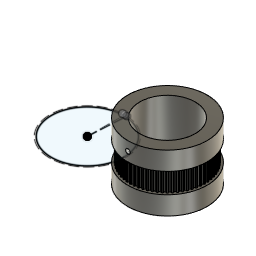
engranaje_gt2_parametrico_torreta (Autodesk Fusion 360 design; units mm, degrees)
Autodesk Fusion 360 part; units mm, degrees
(part 1 of 2)
sketch "Boceto1" plane through (0, 0, 0) normal (0, 0, 1) x (1, 0, 0)
  circle A0 centre (0, 0) radius 20.3718 construction
  line L0 (0, 0) -> (0, 19.6218) construction
  line L1 (0, 0) -> (0.9996, 20.3473) construction
  line L2 (0, 0) -> (1.3989, 20.3237) construction
  arc A1 (0.4973, 19.8971) -> (0.9628, 19.5982) centre (0.99, 20.1525) ccw
  arc A2 (0.2554, 20.3702) -> (0, 20.3718) centre (0, 0) ccw
  arc A3 (0.403, 20.2337) -> (0.2554, 20.3702) centre (0.2536, 20.2202) ccw
  arc A4 (0.403, 20.2337) -> (0.444, 20.0269) centre (1.3989, 20.3237) ccw
  arc A5 (0.444, 20.0269) -> (0.4973, 19.8971) centre (1.2025, 20.2627) ccw
  arc A6 (0, 20.3718) -> (-0.2554, 20.3702) centre (0, 0) ccw
  arc A7 (-0.2554, 20.3702) -> (-0.403, 20.2337) centre (-0.2536, 20.2202) ccw
  arc A8 (-0.444, 20.0269) -> (-0.403, 20.2337) centre (-1.3989, 20.3237) ccw
  arc A9 (-0.4973, 19.8971) -> (-0.444, 20.0269) centre (-1.2025, 20.2627) ccw
  arc A10 (-0.9628, 19.5982) -> (-0.4973, 19.8971) centre (-0.99, 20.1525) ccw
  arc A11 (0.9628, 19.5982) -> (-0.9628, 19.5982) centre (0, 0) ccw construction
  arc A12 (0.9628, 19.5982) -> (-0.9628, 19.5982) centre (0, 0) ccw
  circle A13 centre (0, 0) radius 19.6218
  dimension "d21" = 2.812
  dimension "d22" = 1.125
  dimension "d23" = 0.75
  dimension "d24" = 40.7437
  dimension "d25" = 0.555
  dimension "d26" = 2
  dimension "d27" = 0.3
  dimension "d31" = 0.75
  constraint coincident A0.centre L0.start
  constraint coincident L0.end A11
  constraint vertical L0
  constraint coincident A0 L1.end
  constraint coincident A0 L2.end
  constraint coincident L1 A1.end
  constraint coincident L1 A1.centre
  constraint coincident L2.end A4.centre
  constraint tangent A3 A4
  constraint tangent A0 A3
  constraint coincident A0 A2.end
  constraint tangent A4 A5
  constraint tangent A1 A5
  constraint symmetric L0 A1.start A9.start
  constraint symmetric L0 A1.end A10.start
  constraint symmetric L0 A1 A10
  constraint symmetric L0 A2.start A6.end
  constraint symmetric L0 A2.end A6.start
  constraint symmetric L0 A2 A6
  constraint symmetric L0 A3.start A7.end
  constraint symmetric L0 A3 A7
  constraint symmetric L0 A4.end A8.start
  constraint symmetric L0 A4 A8
  constraint symmetric L0 A5 A9
  constraint concentric A0 A12
  constraint coincident L0.end A12
  constraint concentric A12 A13
  measures "d21" angle of L0 L1
  measures "d22" angle of L1 L2
  measures "d23" distance of A0 A11
  measures "d24" diameter of A0
  measures "d25" radius of A1
  measures "d26" diameter of A4
  measures "d27" diameter of A3
  measures "d31" distance of A0 A13
sketch "Boceto5" plane through (0, 0, 0) normal (0, 0, 1) x (1, 0, 0)
sketch "Boceto6" plane through (0, 0, 0) normal (0, 0, 1) x (1, 0, 0)
sketch "Boceto7" plane through (0, 0, 0) normal (0, 0, 1) x (1, 0, 0)
extrude "Extruir8" add sketch "Boceto1" along normal blind 11 contours A1 A2 A3 A4 A5 A6 A7 A8 A9 A10 A12 A13 makes body 1
pattern_circular "Patrón C3" count 64 over 360 about axis through (0, 0, 1.75) along (0, 0, 1) of bodies 1 makes body 2 at (-2.6672, 19.4397, 7.3333) makes body 3 at (-4.5598, 19.0847, 7.3333) makes body 4 at (-6.4085, 18.5458, 7.3333) makes body 5 at (-7.6077, 18.087, 7.3333) makes body 6 at (-9.3439, 17.2542, 7.3333) makes body 7 at (-10.2706, 16.7192, 3.6667) makes body 8 at (-13.0178, 14.6817, 7.3333) makes body 9 at (-14.3942, 13.335, 7.3333) makes body 10 at (-15.632, 11.8599, 7.3333) makes body 11 at (-15.887, 11.5161, 3.6667) makes body 12 at (-17.5507, 8.7744, 7.3333) makes body 13 at (-18.1689, 7.41, 7.3333) makes body 14 at (-18.5458, 6.4085, 3.6667) makes body 15 at (-19.3769, 3.0907, 7.3333) makes body 16 at (-19.5865, 1.1765, 7.3333) makes body 17 at (-19.6075, 0.749, 3.6667) makes body 18 at (-19.4397, -2.6672, 7.3333) makes body 19 at (-19.3769, -3.0907, 3.6667) makes body 20 at (-18.7456, -5.7982, 7.3333) makes body 21 at (-18.087, -7.6077, 7.3333) makes body 22 at (-16.9392, -9.9035, 7.3333) makes body 23 at (-16.2553, -10.9901, 7.3333) makes body 24 at (-14.6817, -13.0178, 7.3333) makes body 25 at (-14.3942, -13.335, 3.6667) makes body 26 at (-11.8599, -15.632, 7.3333) makes body 27 at (-10.8122, -16.3742, 7.3333) makes body 28 at (-9.1551, -17.3551, 7.3333) makes body 29 at (-7.41, -18.1689, 7.3333) makes body 30 at (-6.4085, -18.5458, 3.6667) makes body 31 at (-3.0907, -19.3769, 7.3333) makes body 32 at (-1.1765, -19.5865, 7.3333) makes body 33 at (-0.749, -19.6075, 3.6667) makes body 34 at (2.6672, -19.4397, 7.3333) makes body 35 at (3.0907, -19.3769, 3.6667) makes body 36 at (6.4085, -18.5458, 7.3333) makes body 37 at (8.1954, -17.8284, 7.3333) makes body 38 at (8.5824, -17.6454, 3.6667) makes body 39 at (11.3421, -16.0116, 7.3333) makes body 40 at (13.0178, -14.6817, 7.3333) makes body 41 at (13.335, -14.3942, 3.6667) makes body 42 at (15.632, -11.8599, 7.3333) makes body 43 at (15.887, -11.5161, 3.6667) makes body 44 at (17.6454, -8.5824, 7.3333) makes body 45 at (18.1689, -7.41, 7.3333) makes body 46 at (18.5458, -6.4085, 3.6667) makes body 47 at (19.3769, -3.0907, 7.3333) makes body 48 at (19.5865, -1.1765, 7.3333) makes body 49 at (19.6075, 0.749, 7.3333) makes body 50 at (19.4397, 2.6672, 7.3333) makes body 51 at (19.3769, 3.0907, 3.6667) makes body 52 at (18.5458, 6.4085, 7.3333) makes body 53 at (18.087, 7.6077, 7.3333) makes body 54 at (17.2542, 9.3439, 7.3333) makes body 55 at (16.2553, 10.9901, 7.3333) makes body 56 at (14.6817, 13.0178, 7.3333) makes body 57 at (13.335, 14.3942, 7.3333) makes body 58 at (11.8599, 15.632, 7.3333) makes body 59 at (11.5161, 15.887, 3.6667) makes body 60 at (8.5824, 17.6454, 7.3333) makes body 61 at (7.41, 18.1689, 7.3333) makes body 62 at (6.4085, 18.5458, 3.6667) makes body 63 at (3.723, 19.2654, 7.3333) makes body 64 at (1.1765, 19.5865, 7.3333)
extrude "Extruir9" add sketch "Boceto1" along normal blind 11 contours A12 A13 bodies 1 2 3 4 5 6 7 8 9 10 11 12 13 14 15 16 17 18 19 20 21 22 23 24 25 26 27 28 29 30 31 32 33 34 35 36 37 38 39 40 41 42 43 44 45 46 47 48 49 50 51 52 53 54 55 56 57 58 59 60 61 62 63 64
sketch "Boceto8" plane through (0, 0, 11) normal (0, 0, 1) x (-1, 0, 0)
  arc A0 (0.403, 20.2337) -> (0.2554, 20.3702) centre (0.2536, 20.2202) ccw
  arc A1 (0.2554, 20.3702) -> (-0.2554, 20.3702) centre (0, 0) ccw
  arc A2 (-0.2554, 20.3702) -> (-0.403, 20.2337) centre (-0.2536, 20.2202) ccw
  arc A3 (-0.444, 20.0269) -> (-0.403, 20.2337) centre (-1.3989, 20.3237) ccw
  arc A4 (-0.4973, 19.8971) -> (-0.444, 20.0269) centre (-1.2025, 20.2627) ccw
  arc A5 (-0.9628, 19.5982) -> (-0.4973, 19.8971) centre (-0.99, 20.1525) ccw
  arc A6 (-1.4553, 19.85) -> (-0.9628, 19.5982) centre (-0.99, 20.1525) ccw
  arc A7 (-1.5211, 19.974) -> (-1.4553, 19.85) centre (-0.7893, 20.283) ccw
  arc A8 (-1.5822, 20.1758) -> (-1.5211, 19.974) centre (-0.5999, 20.363) ccw
  arc A9 (-1.5822, 20.1758) -> (-1.7424, 20.2972) centre (-1.7296, 20.1477) ccw
  arc A10 (-1.7424, 20.2972) -> (-2.2508, 20.2471) centre (0, 0) ccw
  arc A11 (-2.2508, 20.2471) -> (-2.3843, 20.0968) centre (-2.2343, 20.098) ccw
  arc A12 (-2.4048, 19.887) -> (-2.3843, 20.0968) centre (-3.3842, 20.0888) ccw
  arc A13 (-2.4452, 19.7525) -> (-2.4048, 19.887) centre (-3.1828, 20.0473) ccw
  arc A14 (-2.8791, 19.4095) -> (-2.4452, 19.7525) centre (-2.9606, 19.9584) ccw
  arc A15 (-3.394, 19.6118) -> (-2.8791, 19.4095) centre (-2.9606, 19.9584) ccw
  arc A16 (-3.4716, 19.7287) -> (-3.394, 19.6118) centre (-2.7736, 20.108) ccw
  arc A17 (-3.5522, 19.9236) -> (-3.4716, 19.7287) centre (-2.5929, 20.2061) ccw
  arc A18 (-3.5522, 19.9236) -> (-3.7235, 20.0287) centre (-3.6961, 19.8812) ccw
  arc A19 (-3.7235, 20.0287) -> (-4.2245, 19.929) centre (0, 0) ccw
  arc A20 (-4.2245, 19.929) -> (-4.3426, 19.7663) centre (-4.1935, 19.7822) ccw
  arc A21 (-4.3425, 19.5555) -> (-4.3426, 19.7663) centre (-5.337, 19.6603) ccw
  arc A22 (-4.3695, 19.4177) -> (-4.3425, 19.5555) centre (-5.1325, 19.6388) ccw
  arc A23 (-4.7677, 19.0338) -> (-4.3695, 19.4177) centre (-4.9026, 19.5722) ccw
  arc A24 (-5.2999, 19.1847) -> (-4.7677, 19.0338) centre (-4.9026, 19.5722) ccw
  arc A25 (-5.3886, 19.2934) -> (-5.2999, 19.1847) centre (-4.7312, 19.7393) ccw
  arc A26 (-5.4879, 19.4795) -> (-5.3886, 19.2934) centre (-4.561, 19.8547) ccw
  arc A27 (-5.4879, 19.4795) -> (-5.6687, 19.5672) centre (-5.627, 19.4232) ccw
  arc A28 (-5.6687, 19.5672) -> (-6.1576, 19.419) centre (0, 0) ccw
  arc A29 (-6.1576, 19.419) -> (-6.2592, 19.2455) centre (-6.1123, 19.276) ccw
  arc A30 (-6.2384, 19.0357) -> (-6.2592, 19.2455) centre (-7.2383, 19.0425) ccw
  arc A31 (-6.2517, 18.896) -> (-6.2384, 19.0357) centre (-7.0327, 19.0411) ccw
  arc A32 (-6.6104, 18.4748) -> (-6.2517, 18.896) centre (-6.7974, 18.9974) ccw
  arc A33 (-7.1548, 18.5728) -> (-6.6104, 18.4748) centre (-6.7974, 18.9974) ccw
  arc A34 (-7.2538, 18.6723) -> (-7.1548, 18.5728) centre (-6.6432, 19.1805) ccw
  arc A35 (-7.3708, 18.8477) -> (-7.2538, 18.6723) centre (-6.4851, 19.312) ccw
  arc A36 (-7.3708, 18.8477) -> (-7.5594, 18.9174) centre (-7.5037, 18.7781) ccw
  arc A37 (-7.5594, 18.9174) -> (-8.0313, 18.7219) centre (0, 0) ccw
  arc A38 (-8.0313, 18.7219) -> (-8.1154, 18.5393) centre (-7.9722, 18.584) ccw
  arc A39 (-8.0741, 18.3325) -> (-8.1154, 18.5393) centre (-9.07, 18.2414) ccw
  arc A40 (-8.0737, 18.1922) -> (-8.0741, 18.3325) centre (-8.8652, 18.2601) ccw
  arc A41 (-8.3894, 17.7379) -> (-8.0737, 18.1922) centre (-8.6267, 18.2396) ccw
  arc A42 (-8.9408, 17.7821) -> (-8.3894, 17.7379) centre (-8.6267, 18.2396) ccw
  arc A43 (-9.0491, 17.8714) -> (-8.9408, 17.7821) centre (-8.4912, 18.437) ccw
  arc A44 (-9.1827, 18.0345) -> (-9.0491, 17.8714) centre (-8.3468, 18.5834) ccw
  arc A45 (-9.1827, 18.0345) -> (-9.3772, 18.0853) centre (-9.3081, 17.9522) ccw
  arc A46 (-9.3772, 18.0853) -> (-9.8277, 17.8445) centre (0, 0) ccw
  arc A47 (-9.8277, 17.8445) -> (-9.8935, 17.6546) centre (-9.7554, 17.7131) ccw
  arc A48 (-9.8322, 17.4529) -> (-9.8935, 17.6546) centre (-10.8143, 17.2645) ccw
  arc A49 (-9.818, 17.3132) -> (-9.8322, 17.4529) centre (-10.6123, 17.3032) ccw
  arc A50 (-10.0876, 16.8302) -> (-9.818, 17.3132) centre (-10.373, 17.3062) ccw
  arc A51 (-10.6407, 16.8201) -> (-10.0876, 16.8302) centre (-10.373, 17.3062) ccw
  arc A52 (-10.7572, 16.8984) -> (-10.6407, 16.8201) centre (-10.2575, 17.5159) ccw
  arc A53 (-10.9062, 17.0476) -> (-10.7572, 16.8984) centre (-10.1281, 17.6758) ccw
  arc A54 (-10.9062, 17.0476) -> (-11.1047, 17.0791) centre (-11.0229, 16.9534) ccw
  arc A55 (-11.1047, 17.0791) -> (-11.5295, 16.7953) centre (0, 0) ccw
  arc A56 (-11.5295, 16.7953) -> (-11.5763, 16.5999) centre (-11.4446, 16.6716) ccw
  arc A57 (-11.4955, 16.4051) -> (-11.5763, 16.5999) centre (-12.4544, 16.1214) ccw
  arc A58 (-11.4677, 16.2675) -> (-11.4955, 16.4051) centre (-12.2572, 16.1797) ccw
  arc A59 (-11.6887, 15.7604) -> (-11.4677, 16.2675) centre (-12.0193, 16.2062) ccw
  arc A60 (-12.2381, 15.6961) -> (-11.6887, 15.7604) centre (-12.0193, 16.2062) ccw
  arc A61 (-12.3617, 15.7627) -> (-12.2381, 15.6961) centre (-11.9249, 16.4262) ccw
  arc A62 (-12.5247, 15.8965) -> (-12.3617, 15.7627) centre (-11.8119, 16.5979) ccw
  arc A63 (-12.5247, 15.8965) -> (-12.7253, 15.9084) centre (-12.6316, 15.7913) ccw
  arc A64 (-12.7253, 15.9084) -> (-13.1202, 15.5844) centre (0, 0) ccw
  arc A65 (-13.1202, 15.5844) -> (-13.1476, 15.3853) centre (-13.0236, 15.4696) ccw
  arc A66 (-13.0481, 15.1994) -> (-13.1476, 15.3853) centre (-13.9746, 14.823) ccw
  arc A67 (-13.007, 15.0652) -> (-13.0481, 15.1994) centre (-13.7841, 14.9004) ccw
  arc A68 (-13.1772, 14.5388) -> (-13.007, 15.0652) centre (-13.5499, 14.95) ccw
  arc A69 (-13.7177, 14.421) -> (-13.1772, 14.5388) centre (-13.5499, 14.95) ccw
  arc A70 (-13.8472, 14.4751) -> (-13.7177, 14.421) centre (-13.4776, 15.1782) ccw
  arc A71 (-14.0225, 14.5924) -> (-13.8472, 14.4751) centre (-13.3819, 15.3602) ccw
  arc A72 (-14.0225, 14.5924) -> (-14.2233, 14.5845) centre (-14.1186, 14.4772) ccw
  arc A73 (-14.2233, 14.5845) -> (-14.5845, 14.2233) centre (0, 0) ccw
  arc A74 (-14.5845, 14.2233) -> (-14.5924, 14.0225) centre (-14.4772, 14.1186) ccw
  arc A75 (-14.4751, 13.8472) -> (-14.5924, 14.0225) centre (-15.3602, 13.3819) ccw
  arc A76 (-14.421, 13.7177) -> (-14.4751, 13.8472) centre (-15.1782, 13.4776) ccw
  arc A77 (-14.5388, 13.1772) -> (-14.421, 13.7177) centre (-14.95, 13.5499) ccw
  arc A78 (-15.0652, 13.007) -> (-14.5388, 13.1772) centre (-14.95, 13.5499) ccw
  arc A79 (-15.1994, 13.0481) -> (-15.0652, 13.007) centre (-14.9004, 13.7841) ccw
  arc A80 (-15.3853, 13.1476) -> (-15.1994, 13.0481) centre (-14.823, 13.9746) ccw
  arc A81 (-15.3853, 13.1476) -> (-15.5844, 13.1202) centre (-15.4696, 13.0236) ccw
  arc A82 (-15.5844, 13.1202) -> (-15.9084, 12.7253) centre (0, 0) ccw
  arc A83 (-15.9084, 12.7253) -> (-15.8965, 12.5247) centre (-15.7913, 12.6316) ccw
  arc A84 (-15.7627, 12.3617) -> (-15.8965, 12.5247) centre (-16.5979, 11.8119) ccw
  arc A85 (-15.6961, 12.2381) -> (-15.7627, 12.3617) centre (-16.4262, 11.9249) ccw
  arc A86 (-15.7604, 11.6887) -> (-15.6961, 12.2381) centre (-16.2062, 12.0193) ccw
  arc A87 (-16.2675, 11.4677) -> (-15.7604, 11.6887) centre (-16.2062, 12.0193) ccw
  arc A88 (-16.4051, 11.4955) -> (-16.2675, 11.4677) centre (-16.1797, 12.2572) ccw
  arc A89 (-16.5999, 11.5763) -> (-16.4051, 11.4955) centre (-16.1214, 12.4544) ccw
  arc A90 (-16.5999, 11.5763) -> (-16.7953, 11.5295) centre (-16.6716, 11.4446) ccw
  arc A91 (-16.7953, 11.5295) -> (-17.0791, 11.1047) centre (0, 0) ccw
  arc A92 (-17.0791, 11.1047) -> (-17.0476, 10.9062) centre (-16.9534, 11.0229) ccw
  arc A93 (-16.8984, 10.7572) -> (-17.0476, 10.9062) centre (-17.6758, 10.1281) ccw
  arc A94 (-16.8201, 10.6407) -> (-16.8984, 10.7572) centre (-17.5159, 10.2575) ccw
  arc A95 (-16.8302, 10.0876) -> (-16.8201, 10.6407) centre (-17.3062, 10.373) ccw
  arc A96 (-17.3132, 9.818) -> (-16.8302, 10.0876) centre (-17.3062, 10.373) ccw
  arc A97 (-17.4529, 9.8322) -> (-17.3132, 9.818) centre (-17.3032, 10.6123) ccw
  arc A98 (-17.6546, 9.8935) -> (-17.4529, 9.8322) centre (-17.2645, 10.8143) ccw
  arc A99 (-17.6546, 9.8935) -> (-17.8445, 9.8277) centre (-17.7131, 9.7554) ccw
  arc A100 (-17.8445, 9.8277) -> (-18.0853, 9.3772) centre (0, 0) ccw
  arc A101 (-18.0853, 9.3772) -> (-18.0345, 9.1827) centre (-17.9522, 9.3081) ccw
  arc A102 (-17.8714, 9.0491) -> (-18.0345, 9.1827) centre (-18.5834, 8.3468) ccw
  arc A103 (-17.7821, 8.9408) -> (-17.8714, 9.0491) centre (-18.437, 8.4912) ccw
  arc A104 (-17.7379, 8.3894) -> (-17.7821, 8.9408) centre (-18.2396, 8.6267) ccw
  arc A105 (-18.1922, 8.0737) -> (-17.7379, 8.3894) centre (-18.2396, 8.6267) ccw
  arc A106 (-18.3325, 8.0741) -> (-18.1922, 8.0737) centre (-18.2601, 8.8652) ccw
  arc A107 (-18.5393, 8.1154) -> (-18.3325, 8.0741) centre (-18.2414, 9.07) ccw
  arc A108 (-18.5393, 8.1154) -> (-18.7219, 8.0313) centre (-18.584, 7.9722) ccw
  arc A109 (-18.7219, 8.0313) -> (-18.9174, 7.5594) centre (0, 0) ccw
  arc A110 (-18.9174, 7.5594) -> (-18.8477, 7.3708) centre (-18.7781, 7.5037) ccw
  arc A111 (-18.6723, 7.2538) -> (-18.8477, 7.3708) centre (-19.312, 6.4851) ccw
  arc A112 (-18.5728, 7.1548) -> (-18.6723, 7.2538) centre (-19.1805, 6.6432) ccw
  arc A113 (-18.4748, 6.6104) -> (-18.5728, 7.1548) centre (-18.9974, 6.7974) ccw
  arc A114 (-18.896, 6.2517) -> (-18.4748, 6.6104) centre (-18.9974, 6.7974) ccw
  arc A115 (-19.0357, 6.2384) -> (-18.896, 6.2517) centre (-19.0411, 7.0327) ccw
  arc A116 (-19.2455, 6.2592) -> (-19.0357, 6.2384) centre (-19.0425, 7.2383) ccw
  arc A117 (-19.2455, 6.2592) -> (-19.419, 6.1576) centre (-19.276, 6.1123) ccw
  arc A118 (-19.419, 6.1576) -> (-19.5672, 5.6687) centre (0, 0) ccw
  arc A119 (-19.5672, 5.6687) -> (-19.4795, 5.4879) centre (-19.4232, 5.627) ccw
  arc A120 (-19.2934, 5.3886) -> (-19.4795, 5.4879) centre (-19.8547, 4.561) ccw
  arc A121 (-19.1847, 5.2999) -> (-19.2934, 5.3886) centre (-19.7393, 4.7312) ccw
  arc A122 (-19.0338, 4.7677) -> (-19.1847, 5.2999) centre (-19.5722, 4.9026) ccw
  arc A123 (-19.4177, 4.3695) -> (-19.0338, 4.7677) centre (-19.5722, 4.9026) ccw
  arc A124 (-19.5555, 4.3425) -> (-19.4177, 4.3695) centre (-19.6388, 5.1325) ccw
  arc A125 (-19.7663, 4.3426) -> (-19.5555, 4.3425) centre (-19.6603, 5.337) ccw
  arc A126 (-19.7663, 4.3426) -> (-19.929, 4.2245) centre (-19.7822, 4.1935) ccw
  arc A127 (-19.929, 4.2245) -> (-20.0287, 3.7235) centre (0, 0) ccw
  arc A128 (-20.0287, 3.7235) -> (-19.9236, 3.5522) centre (-19.8812, 3.6961) ccw
  arc A129 (-19.7287, 3.4716) -> (-19.9236, 3.5522) centre (-20.2061, 2.5929) ccw
  arc A130 (-19.6118, 3.394) -> (-19.7287, 3.4716) centre (-20.108, 2.7736) ccw
  arc A131 (-19.4095, 2.8791) -> (-19.6118, 3.394) centre (-19.9584, 2.9606) ccw
  arc A132 (-19.7525, 2.4452) -> (-19.4095, 2.8791) centre (-19.9584, 2.9606) ccw
  arc A133 (-19.887, 2.4048) -> (-19.7525, 2.4452) centre (-20.0473, 3.1828) ccw
  arc A134 (-20.0968, 2.3843) -> (-19.887, 2.4048) centre (-20.0888, 3.3842) ccw
  arc A135 (-20.0968, 2.3843) -> (-20.2471, 2.2508) centre (-20.098, 2.2343) ccw
  arc A136 (-20.2471, 2.2508) -> (-20.2972, 1.7424) centre (0, 0) ccw
  arc A137 (-20.2972, 1.7424) -> (-20.1758, 1.5822) centre (-20.1477, 1.7296) ccw
  arc A138 (-19.974, 1.5211) -> (-20.1758, 1.5822) centre (-20.363, 0.5999) ccw
  arc A139 (-19.85, 1.4553) -> (-19.974, 1.5211) centre (-20.283, 0.7893) ccw
  arc A140 (-19.5982, 0.9628) -> (-19.85, 1.4553) centre (-20.1525, 0.99) ccw
  arc A141 (-19.8971, 0.4973) -> (-19.5982, 0.9628) centre (-20.1525, 0.99) ccw
  arc A142 (-20.0269, 0.444) -> (-19.8971, 0.4973) centre (-20.2627, 1.2025) ccw
  arc A143 (-20.2337, 0.403) -> (-20.0269, 0.444) centre (-20.3237, 1.3989) ccw
  arc A144 (-20.2337, 0.403) -> (-20.3702, 0.2554) centre (-20.2202, 0.2536) ccw
  arc A145 (-20.3702, 0.2554) -> (-20.3702, -0.2554) centre (0, 0) ccw
  arc A146 (-20.3702, -0.2554) -> (-20.2337, -0.403) centre (-20.2202, -0.2536) ccw
  arc A147 (-20.0269, -0.444) -> (-20.2337, -0.403) centre (-20.3237, -1.3989) ccw
  arc A148 (-19.8971, -0.4973) -> (-20.0269, -0.444) centre (-20.2627, -1.2025) ccw
  arc A149 (-19.5982, -0.9628) -> (-19.8971, -0.4973) centre (-20.1525, -0.99) ccw
  arc A150 (-19.85, -1.4553) -> (-19.5982, -0.9628) centre (-20.1525, -0.99) ccw
  arc A151 (-19.974, -1.5211) -> (-19.85, -1.4553) centre (-20.283, -0.7893) ccw
  arc A152 (-20.1758, -1.5822) -> (-19.974, -1.5211) centre (-20.363, -0.5999) ccw
  arc A153 (-20.1758, -1.5822) -> (-20.2972, -1.7424) centre (-20.1477, -1.7296) ccw
  arc A154 (-20.2972, -1.7424) -> (-20.2471, -2.2508) centre (0, 0) ccw
  arc A155 (-20.2471, -2.2508) -> (-20.0968, -2.3843) centre (-20.098, -2.2343) ccw
  arc A156 (-19.887, -2.4048) -> (-20.0968, -2.3843) centre (-20.0888, -3.3842) ccw
  arc A157 (-19.7525, -2.4452) -> (-19.887, -2.4048) centre (-20.0473, -3.1828) ccw
  arc A158 (-19.4095, -2.8791) -> (-19.7525, -2.4452) centre (-19.9584, -2.9606) ccw
  arc A159 (-19.6118, -3.394) -> (-19.4095, -2.8791) centre (-19.9584, -2.9606) ccw
  arc A160 (-19.7287, -3.4716) -> (-19.6118, -3.394) centre (-20.108, -2.7736) ccw
  arc A161 (-19.9236, -3.5522) -> (-19.7287, -3.4716) centre (-20.2061, -2.5929) ccw
  arc A162 (-19.9236, -3.5522) -> (-20.0287, -3.7235) centre (-19.8812, -3.6961) ccw
  arc A163 (-20.0287, -3.7235) -> (-19.929, -4.2245) centre (0, 0) ccw
  arc A164 (-19.929, -4.2245) -> (-19.7663, -4.3426) centre (-19.7822, -4.1935) ccw
  arc A165 (-19.5555, -4.3425) -> (-19.7663, -4.3426) centre (-19.6603, -5.337) ccw
  arc A166 (-19.4177, -4.3695) -> (-19.5555, -4.3425) centre (-19.6388, -5.1325) ccw
  arc A167 (-19.0338, -4.7677) -> (-19.4177, -4.3695) centre (-19.5722, -4.9026) ccw
  arc A168 (-19.1847, -5.2999) -> (-19.0338, -4.7677) centre (-19.5722, -4.9026) ccw
  arc A169 (-19.2934, -5.3886) -> (-19.1847, -5.2999) centre (-19.7393, -4.7312) ccw
  arc A170 (-19.4795, -5.4879) -> (-19.2934, -5.3886) centre (-19.8547, -4.561) ccw
  arc A171 (-19.4795, -5.4879) -> (-19.5672, -5.6687) centre (-19.4232, -5.627) ccw
  arc A172 (-19.5672, -5.6687) -> (-19.419, -6.1576) centre (0, 0) ccw
  arc A173 (-19.419, -6.1576) -> (-19.2455, -6.2592) centre (-19.276, -6.1123) ccw
  arc A174 (-19.0357, -6.2384) -> (-19.2455, -6.2592) centre (-19.0425, -7.2383) ccw
  arc A175 (-18.896, -6.2517) -> (-19.0357, -6.2384) centre (-19.0411, -7.0327) ccw
  arc A176 (-18.4748, -6.6104) -> (-18.896, -6.2517) centre (-18.9974, -6.7974) ccw
  arc A177 (-18.5728, -7.1548) -> (-18.4748, -6.6104) centre (-18.9974, -6.7974) ccw
  arc A178 (-18.6723, -7.2538) -> (-18.5728, -7.1548) centre (-19.1805, -6.6432) ccw
  arc A179 (-18.8477, -7.3708) -> (-18.6723, -7.2538) centre (-19.312, -6.4851) ccw
  arc A180 (-18.8477, -7.3708) -> (-18.9174, -7.5594) centre (-18.7781, -7.5037) ccw
  arc A181 (-18.9174, -7.5594) -> (-18.7219, -8.0313) centre (0, 0) ccw
  arc A182 (-18.7219, -8.0313) -> (-18.5393, -8.1154) centre (-18.584, -7.9722) ccw
  arc A183 (-18.3325, -8.0741) -> (-18.5393, -8.1154) centre (-18.2414, -9.07) ccw
  arc A184 (-18.1922, -8.0737) -> (-18.3325, -8.0741) centre (-18.2601, -8.8652) ccw
  arc A185 (-17.7379, -8.3894) -> (-18.1922, -8.0737) centre (-18.2396, -8.6267) ccw
  arc A186 (-17.7821, -8.9408) -> (-17.7379, -8.3894) centre (-18.2396, -8.6267) ccw
  arc A187 (-17.8714, -9.0491) -> (-17.7821, -8.9408) centre (-18.437, -8.4912) ccw
  arc A188 (-18.0345, -9.1827) -> (-17.8714, -9.0491) centre (-18.5834, -8.3468) ccw
  arc A189 (-18.0345, -9.1827) -> (-18.0853, -9.3772) centre (-17.9522, -9.3081) ccw
  arc A190 (-18.0853, -9.3772) -> (-17.8445, -9.8277) centre (0, 0) ccw
  arc A191 (-17.8445, -9.8277) -> (-17.6546, -9.8935) centre (-17.7131, -9.7554) ccw
  arc A192 (-17.4529, -9.8322) -> (-17.6546, -9.8935) centre (-17.2645, -10.8143) ccw
  arc A193 (-17.3132, -9.818) -> (-17.4529, -9.8322) centre (-17.3032, -10.6123) ccw
  arc A194 (-16.8302, -10.0876) -> (-17.3132, -9.818) centre (-17.3062, -10.373) ccw
  arc A195 (-16.8201, -10.6407) -> (-16.8302, -10.0876) centre (-17.3062, -10.373) ccw
  arc A196 (-16.8984, -10.7572) -> (-16.8201, -10.6407) centre (-17.5159, -10.2575) ccw
  arc A197 (-17.0476, -10.9062) -> (-16.8984, -10.7572) centre (-17.6758, -10.1281) ccw
  arc A198 (-17.0476, -10.9062) -> (-17.0791, -11.1047) centre (-16.9534, -11.0229) ccw
  arc A199 (-17.0791, -11.1047) -> (-16.7953, -11.5295) centre (0, 0) ccw
  arc A200 (-16.7953, -11.5295) -> (-16.5999, -11.5763) centre (-16.6716, -11.4446) ccw
  arc A201 (-16.4051, -11.4955) -> (-16.5999, -11.5763) centre (-16.1214, -12.4544) ccw
  arc A202 (-16.2675, -11.4677) -> (-16.4051, -11.4955) centre (-16.1797, -12.2572) ccw
  arc A203 (-15.7604, -11.6887) -> (-16.2675, -11.4677) centre (-16.2062, -12.0193) ccw
  arc A204 (-15.6961, -12.2381) -> (-15.7604, -11.6887) centre (-16.2062, -12.0193) ccw
  arc A205 (-15.7627, -12.3617) -> (-15.6961, -12.2381) centre (-16.4262, -11.9249) ccw
  arc A206 (-15.8965, -12.5247) -> (-15.7627, -12.3617) centre (-16.5979, -11.8119) ccw
  arc A207 (-15.8965, -12.5247) -> (-15.9084, -12.7253) centre (-15.7913, -12.6316) ccw
  arc A208 (-15.9084, -12.7253) -> (-15.5844, -13.1202) centre (0, 0) ccw
  arc A209 (-15.5844, -13.1202) -> (-15.3853, -13.1476) centre (-15.4696, -13.0236) ccw
  arc A210 (-15.1994, -13.0481) -> (-15.3853, -13.1476) centre (-14.823, -13.9746) ccw
  arc A211 (-15.0652, -13.007) -> (-15.1994, -13.0481) centre (-14.9004, -13.7841) ccw
  arc A212 (-14.5388, -13.1772) -> (-15.0652, -13.007) centre (-14.95, -13.5499) ccw
  arc A213 (-14.421, -13.7177) -> (-14.5388, -13.1772) centre (-14.95, -13.5499) ccw
  arc A214 (-14.4751, -13.8472) -> (-14.421, -13.7177) centre (-15.1782, -13.4776) ccw
  arc A215 (-14.5924, -14.0225) -> (-14.4751, -13.8472) centre (-15.3602, -13.3819) ccw
  arc A216 (-14.5924, -14.0225) -> (-14.5845, -14.2233) centre (-14.4772, -14.1186) ccw
  arc A217 (-14.5845, -14.2233) -> (-14.2233, -14.5845) centre (0, 0) ccw
  arc A218 (-14.2233, -14.5845) -> (-14.0225, -14.5924) centre (-14.1186, -14.4772) ccw
  arc A219 (-13.8472, -14.4751) -> (-14.0225, -14.5924) centre (-13.3819, -15.3602) ccw
  arc A220 (-13.7177, -14.421) -> (-13.8472, -14.4751) centre (-13.4776, -15.1782) ccw
  arc A221 (-13.1772, -14.5388) -> (-13.7177, -14.421) centre (-13.5499, -14.95) ccw
  arc A222 (-13.007, -15.0652) -> (-13.1772, -14.5388) centre (-13.5499, -14.95) ccw
  arc A223 (-13.0481, -15.1994) -> (-13.007, -15.0652) centre (-13.7841, -14.9004) ccw
  arc A224 (-13.1476, -15.3853) -> (-13.0481, -15.1994) centre (-13.9746, -14.823) ccw
  arc A225 (-13.1476, -15.3853) -> (-13.1202, -15.5844) centre (-13.0236, -15.4696) ccw
  arc A226 (-13.1202, -15.5844) -> (-12.7253, -15.9084) centre (0, 0) ccw
  arc A227 (-12.7253, -15.9084) -> (-12.5247, -15.8965) centre (-12.6316, -15.7913) ccw
  arc A228 (-12.3617, -15.7627) -> (-12.5247, -15.8965) centre (-11.8119, -16.5979) ccw
  arc A229 (-12.2381, -15.6961) -> (-12.3617, -15.7627) centre (-11.9249, -16.4262) ccw
  arc A230 (-11.6887, -15.7604) -> (-12.2381, -15.6961) centre (-12.0193, -16.2062) ccw
  arc A231 (-11.4677, -16.2675) -> (-11.6887, -15.7604) centre (-12.0193, -16.2062) ccw
  arc A232 (-11.4955, -16.4051) -> (-11.4677, -16.2675) centre (-12.2572, -16.1797) ccw
  arc A233 (-11.5763, -16.5999) -> (-11.4955, -16.4051) centre (-12.4544, -16.1214) ccw
  arc A234 (-11.5763, -16.5999) -> (-11.5295, -16.7953) centre (-11.4446, -16.6716) ccw
  arc A235 (-11.5295, -16.7953) -> (-11.1047, -17.0791) centre (0, 0) ccw
  arc A236 (-11.1047, -17.0791) -> (-10.9062, -17.0476) centre (-11.0229, -16.9534) ccw
  arc A237 (-10.7572, -16.8984) -> (-10.9062, -17.0476) centre (-10.1281, -17.6758) ccw
  arc A238 (-10.6407, -16.8201) -> (-10.7572, -16.8984) centre (-10.2575, -17.5159) ccw
  arc A239 (-10.0876, -16.8302) -> (-10.6407, -16.8201) centre (-10.373, -17.3062) ccw
  arc A240 (-9.818, -17.3132) -> (-10.0876, -16.8302) centre (-10.373, -17.3062) ccw
  arc A241 (-9.8322, -17.4529) -> (-9.818, -17.3132) centre (-10.6123, -17.3032) ccw
  arc A242 (-9.8935, -17.6546) -> (-9.8322, -17.4529) centre (-10.8143, -17.2645) ccw
  arc A243 (-9.8935, -17.6546) -> (-9.8277, -17.8445) centre (-9.7554, -17.7131) ccw
  arc A244 (-9.8277, -17.8445) -> (-9.3772, -18.0853) centre (0, 0) ccw
  arc A245 (-9.3772, -18.0853) -> (-9.1827, -18.0345) centre (-9.3081, -17.9522) ccw
  arc A246 (-9.0491, -17.8714) -> (-9.1827, -18.0345) centre (-8.3468, -18.5834) ccw
  arc A247 (-8.9408, -17.7821) -> (-9.0491, -17.8714) centre (-8.4912, -18.437) ccw
  arc A248 (-8.3894, -17.7379) -> (-8.9408, -17.7821) centre (-8.6267, -18.2396) ccw
  arc A249 (-8.0737, -18.1922) -> (-8.3894, -17.7379) centre (-8.6267, -18.2396) ccw
  arc A250 (-8.0741, -18.3325) -> (-8.0737, -18.1922) centre (-8.8652, -18.2601) ccw
  arc A251 (-8.1154, -18.5393) -> (-8.0741, -18.3325) centre (-9.07, -18.2414) ccw
  arc A252 (-8.1154, -18.5393) -> (-8.0313, -18.7219) centre (-7.9722, -18.584) ccw
  arc A253 (-8.0313, -18.7219) -> (-7.5594, -18.9174) centre (0, 0) ccw
  arc A254 (-7.5594, -18.9174) -> (-7.3708, -18.8477) centre (-7.5037, -18.7781) ccw
  arc A255 (-7.2538, -18.6723) -> (-7.3708, -18.8477) centre (-6.4851, -19.312) ccw
  arc A256 (-7.1548, -18.5728) -> (-7.2538, -18.6723) centre (-6.6432, -19.1805) ccw
  arc A257 (-6.6104, -18.4748) -> (-7.1548, -18.5728) centre (-6.7974, -18.9974) ccw
  arc A258 (-6.2517, -18.896) -> (-6.6104, -18.4748) centre (-6.7974, -18.9974) ccw
  arc A259 (-6.2384, -19.0357) -> (-6.2517, -18.896) centre (-7.0327, -19.0411) ccw
  arc A260 (-6.2592, -19.2455) -> (-6.2384, -19.0357) centre (-7.2383, -19.0425) ccw
  arc A261 (-6.2592, -19.2455) -> (-6.1576, -19.419) centre (-6.1123, -19.276) ccw
  arc A262 (-6.1576, -19.419) -> (-5.6687, -19.5672) centre (0, 0) ccw
  arc A263 (-5.6687, -19.5672) -> (-5.4879, -19.4795) centre (-5.627, -19.4232) ccw
  arc A264 (-5.3886, -19.2934) -> (-5.4879, -19.4795) centre (-4.561, -19.8547) ccw
  arc A265 (-5.2999, -19.1847) -> (-5.3886, -19.2934) centre (-4.7312, -19.7393) ccw
  arc A266 (-4.7677, -19.0338) -> (-5.2999, -19.1847) centre (-4.9026, -19.5722) ccw
  arc A267 (-4.3695, -19.4177) -> (-4.7677, -19.0338) centre (-4.9026, -19.5722) ccw
  arc A268 (-4.3425, -19.5555) -> (-4.3695, -19.4177) centre (-5.1325, -19.6388) ccw
  arc A269 (-4.3426, -19.7663) -> (-4.3425, -19.5555) centre (-5.337, -19.6603) ccw
  arc A270 (-4.3426, -19.7663) -> (-4.2245, -19.929) centre (-4.1935, -19.7822) ccw
  arc A271 (-4.2245, -19.929) -> (-3.7235, -20.0287) centre (0, 0) ccw
  arc A272 (-3.7235, -20.0287) -> (-3.5522, -19.9236) centre (-3.6961, -19.8812) ccw
  arc A273 (-3.4716, -19.7287) -> (-3.5522, -19.9236) centre (-2.5929, -20.2061) ccw
  arc A274 (-3.394, -19.6118) -> (-3.4716, -19.7287) centre (-2.7736, -20.108) ccw
  arc A275 (-2.8791, -19.4095) -> (-3.394, -19.6118) centre (-2.9606, -19.9584) ccw
  arc A276 (-2.4452, -19.7525) -> (-2.8791, -19.4095) centre (-2.9606, -19.9584) ccw
  arc A277 (-2.4048, -19.887) -> (-2.4452, -19.7525) centre (-3.1828, -20.0473) ccw
  arc A278 (-2.3843, -20.0968) -> (-2.4048, -19.887) centre (-3.3842, -20.0888) ccw
  arc A279 (-2.3843, -20.0968) -> (-2.2508, -20.2471) centre (-2.2343, -20.098) ccw
  arc A280 (-2.2508, -20.2471) -> (-1.7424, -20.2972) centre (0, 0) ccw
  arc A281 (-1.7424, -20.2972) -> (-1.5822, -20.1758) centre (-1.7296, -20.1477) ccw
  arc A282 (-1.5211, -19.974) -> (-1.5822, -20.1758) centre (-0.5999, -20.363) ccw
  arc A283 (-1.4553, -19.85) -> (-1.5211, -19.974) centre (-0.7893, -20.283) ccw
  arc A284 (-0.9628, -19.5982) -> (-1.4553, -19.85) centre (-0.99, -20.1525) ccw
  arc A285 (-0.4973, -19.8971) -> (-0.9628, -19.5982) centre (-0.99, -20.1525) ccw
  arc A286 (-0.444, -20.0269) -> (-0.4973, -19.8971) centre (-1.2025, -20.2627) ccw
  arc A287 (-0.403, -20.2337) -> (-0.444, -20.0269) centre (-1.3989, -20.3237) ccw
  arc A288 (-0.403, -20.2337) -> (-0.2554, -20.3702) centre (-0.2536, -20.2202) ccw
  arc A289 (-0.2554, -20.3702) -> (0.2554, -20.3702) centre (0, 0) ccw
  arc A290 (0.2554, -20.3702) -> (0.403, -20.2337) centre (0.2536, -20.2202) ccw
  arc A291 (0.444, -20.0269) -> (0.403, -20.2337) centre (1.3989, -20.3237) ccw
  arc A292 (0.4973, -19.8971) -> (0.444, -20.0269) centre (1.2025, -20.2627) ccw
  arc A293 (0.9628, -19.5982) -> (0.4973, -19.8971) centre (0.99, -20.1525) ccw
  arc A294 (1.4553, -19.85) -> (0.9628, -19.5982) centre (0.99, -20.1525) ccw
  arc A295 (1.5211, -19.974) -> (1.4553, -19.85) centre (0.7893, -20.283) ccw
  arc A296 (1.5822, -20.1758) -> (1.5211, -19.974) centre (0.5999, -20.363) ccw
  arc A297 (1.5822, -20.1758) -> (1.7424, -20.2972) centre (1.7296, -20.1477) ccw
  arc A298 (1.7424, -20.2972) -> (2.2508, -20.2471) centre (0, 0) ccw
  arc A299 (2.2508, -20.2471) -> (2.3843, -20.0968) centre (2.2343, -20.098) ccw
  arc A300 (2.4048, -19.887) -> (2.3843, -20.0968) centre (3.3842, -20.0888) ccw
  arc A301 (2.4452, -19.7525) -> (2.4048, -19.887) centre (3.1828, -20.0473) ccw
  arc A302 (2.8791, -19.4095) -> (2.4452, -19.7525) centre (2.9606, -19.9584) ccw
  arc A303 (3.394, -19.6118) -> (2.8791, -19.4095) centre (2.9606, -19.9584) ccw
  arc A304 (3.4716, -19.7287) -> (3.394, -19.6118) centre (2.7736, -20.108) ccw
  arc A305 (3.5522, -19.9236) -> (3.4716, -19.7287) centre (2.5929, -20.2061) ccw
  arc A306 (3.5522, -19.9236) -> (3.7235, -20.0287) centre (3.6961, -19.8812) ccw
  arc A307 (3.7235, -20.0287) -> (4.2245, -19.929) centre (0, 0) ccw
  arc A308 (4.2245, -19.929) -> (4.3426, -19.7663) centre (4.1935, -19.7822) ccw
  arc A309 (4.3425, -19.5555) -> (4.3426, -19.7663) centre (5.337, -19.6603) ccw
  arc A310 (4.3695, -19.4177) -> (4.3425, -19.5555) centre (5.1325, -19.6388) ccw
  arc A311 (4.7677, -19.0338) -> (4.3695, -19.4177) centre (4.9026, -19.5722) ccw
  arc A312 (5.2999, -19.1847) -> (4.7677, -19.0338) centre (4.9026, -19.5722) ccw
  arc A313 (5.3886, -19.2934) -> (5.2999, -19.1847) centre (4.7312, -19.7393) ccw
  arc A314 (5.4879, -19.4795) -> (5.3886, -19.2934) centre (4.561, -19.8547) ccw
  arc A315 (5.4879, -19.4795) -> (5.6687, -19.5672) centre (5.627, -19.4232) ccw
  arc A316 (5.6687, -19.5672) -> (6.1576, -19.419) centre (0, 0) ccw
  arc A317 (6.1576, -19.419) -> (6.2592, -19.2455) centre (6.1123, -19.276) ccw
  arc A318 (6.2384, -19.0357) -> (6.2592, -19.2455) centre (7.2383, -19.0425) ccw
  arc A319 (6.2517, -18.896) -> (6.2384, -19.0357) centre (7.0327, -19.0411) ccw
  arc A320 (6.6104, -18.4748) -> (6.2517, -18.896) centre (6.7974, -18.9974) ccw
  arc A321 (7.1548, -18.5728) -> (6.6104, -18.4748) centre (6.7974, -18.9974) ccw
  arc A322 (7.2538, -18.6723) -> (7.1548, -18.5728) centre (6.6432, -19.1805) ccw
  arc A323 (7.3708, -18.8477) -> (7.2538, -18.6723) centre (6.4851, -19.312) ccw
  arc A324 (7.3708, -18.8477) -> (7.5594, -18.9174) centre (7.5037, -18.7781) ccw
  arc A325 (7.5594, -18.9174) -> (8.0313, -18.7219) centre (0, 0) ccw
  arc A326 (8.0313, -18.7219) -> (8.1154, -18.5393) centre (7.9722, -18.584) ccw
  arc A327 (8.0741, -18.3325) -> (8.1154, -18.5393) centre (9.07, -18.2414) ccw
  arc A328 (8.0737, -18.1922) -> (8.0741, -18.3325) centre (8.8652, -18.2601) ccw
  arc A329 (8.3894, -17.7379) -> (8.0737, -18.1922) centre (8.6267, -18.2396) ccw
  arc A330 (8.9408, -17.7821) -> (8.3894, -17.7379) centre (8.6267, -18.2396) ccw
  arc A331 (9.0491, -17.8714) -> (8.9408, -17.7821) centre (8.4912, -18.437) ccw
  arc A332 (9.1827, -18.0345) -> (9.0491, -17.8714) centre (8.3468, -18.5834) ccw
  arc A333 (9.1827, -18.0345) -> (9.3772, -18.0853) centre (9.3081, -17.9522) ccw
  arc A334 (9.3772, -18.0853) -> (9.8277, -17.8445) centre (0, 0) ccw
  arc A335 (9.8277, -17.8445) -> (9.8935, -17.6546) centre (9.7554, -17.7131) ccw
  arc A336 (9.8322, -17.4529) -> (9.8935, -17.6546) centre (10.8143, -17.2645) ccw
  arc A337 (9.818, -17.3132) -> (9.8322, -17.4529) centre (10.6123, -17.3032) ccw
  arc A338 (10.0876, -16.8302) -> (9.818, -17.3132) centre (10.373, -17.3062) ccw
  arc A339 (10.6407, -16.8201) -> (10.0876, -16.8302) centre (10.373, -17.3062) ccw
  arc A340 (10.7572, -16.8984) -> (10.6407, -16.8201) centre (10.2575, -17.5159) ccw
  arc A341 (10.9062, -17.0476) -> (10.7572, -16.8984) centre (10.1281, -17.6758) ccw
  arc A342 (10.9062, -17.0476) -> (11.1047, -17.0791) centre (11.0229, -16.9534) ccw
  arc A343 (11.1047, -17.0791) -> (11.5295, -16.7953) centre (0, 0) ccw
  arc A344 (11.5295, -16.7953) -> (11.5763, -16.5999) centre (11.4446, -16.6716) ccw
  arc A345 (11.4955, -16.4051) -> (11.5763, -16.5999) centre (12.4544, -16.1214) ccw
  arc A346 (11.4677, -16.2675) -> (11.4955, -16.4051) centre (12.2572, -16.1797) ccw
  arc A347 (11.6887, -15.7604) -> (11.4677, -16.2675) centre (12.0193, -16.2062) ccw
  arc A348 (12.2381, -15.6961) -> (11.6887, -15.7604) centre (12.0193, -16.2062) ccw
  arc A349 (12.3617, -15.7627) -> (12.2381, -15.6961) centre (11.9249, -16.4262) ccw
  arc A350 (12.5247, -15.8965) -> (12.3617, -15.7627) centre (11.8119, -16.5979) ccw
  arc A351 (12.5247, -15.8965) -> (12.7253, -15.9084) centre (12.6316, -15.7913) ccw
  arc A352 (12.7253, -15.9084) -> (13.1202, -15.5844) centre (0, 0) ccw
  arc A353 (13.1202, -15.5844) -> (13.1476, -15.3853) centre (13.0236, -15.4696) ccw
  arc A354 (13.0481, -15.1994) -> (13.1476, -15.3853) centre (13.9746, -14.823) ccw
  arc A355 (13.007, -15.0652) -> (13.0481, -15.1994) centre (13.7841, -14.9004) ccw
  arc A356 (13.1772, -14.5388) -> (13.007, -15.0652) centre (13.5499, -14.95) ccw
  arc A357 (13.7177, -14.421) -> (13.1772, -14.5388) centre (13.5499, -14.95) ccw
  arc A358 (13.8472, -14.4751) -> (13.7177, -14.421) centre (13.4776, -15.1782) ccw
  arc A359 (14.0225, -14.5924) -> (13.8472, -14.4751) centre (13.3819, -15.3602) ccw
  arc A360 (14.0225, -14.5924) -> (14.2233, -14.5845) centre (14.1186, -14.4772) ccw
  arc A361 (14.2233, -14.5845) -> (14.5845, -14.2233) centre (0, 0) ccw
  arc A362 (14.5845, -14.2233) -> (14.5924, -14.0225) centre (14.4772, -14.1186) ccw
  arc A363 (14.4751, -13.8472) -> (14.5924, -14.0225) centre (15.3602, -13.3819) ccw
  arc A364 (14.421, -13.7177) -> (14.4751, -13.8472) centre (15.1782, -13.4776) ccw
  arc A365 (14.5388, -13.1772) -> (14.421, -13.7177) centre (14.95, -13.5499) ccw
  arc A366 (15.0652, -13.007) -> (14.5388, -13.1772) centre (14.95, -13.5499) ccw
  arc A367 (15.1994, -13.0481) -> (15.0652, -13.007) centre (14.9004, -13.7841) ccw
  arc A368 (15.3853, -13.1476) -> (15.1994, -13.0481) centre (14.823, -13.9746) ccw
  arc A369 (15.3853, -13.1476) -> (15.5844, -13.1202) centre (15.4696, -13.0236) ccw
  arc A370 (15.5844, -13.1202) -> (15.9084, -12.7253) centre (0, 0) ccw
  arc A371 (15.9084, -12.7253) -> (15.8965, -12.5247) centre (15.7913, -12.6316) ccw
  arc A372 (15.7627, -12.3617) -> (15.8965, -12.5247) centre (16.5979, -11.8119) ccw
  arc A373 (15.6961, -12.2381) -> (15.7627, -12.3617) centre (16.4262, -11.9249) ccw
  arc A374 (15.7604, -11.6887) -> (15.6961, -12.2381) centre (16.2062, -12.0193) ccw
  arc A375 (16.2675, -11.4677) -> (15.7604, -11.6887) centre (16.2062, -12.0193) ccw
  arc A376 (16.4051, -11.4955) -> (16.2675, -11.4677) centre (16.1797, -12.2572) ccw
  arc A377 (16.5999, -11.5763) -> (16.4051, -11.4955) centre (16.1214, -12.4544) ccw
  arc A378 (16.5999, -11.5763) -> (16.7953, -11.5295) centre (16.6716, -11.4446) ccw
  arc A379 (16.7953, -11.5295) -> (17.0791, -11.1047) centre (0, 0) ccw
  arc A380 (17.0791, -11.1047) -> (17.0476, -10.9062) centre (16.9534, -11.0229) ccw
  arc A381 (16.8984, -10.7572) -> (17.0476, -10.9062) centre (17.6758, -10.1281) ccw
  arc A382 (16.8201, -10.6407) -> (16.8984, -10.7572) centre (17.5159, -10.2575) ccw
  arc A383 (16.8302, -10.0876) -> (16.8201, -10.6407) centre (17.3062, -10.373) ccw
  arc A384 (17.3132, -9.818) -> (16.8302, -10.0876) centre (17.3062, -10.373) ccw
  arc A385 (17.4529, -9.8322) -> (17.3132, -9.818) centre (17.3032, -10.6123) ccw
  arc A386 (17.6546, -9.8935) -> (17.4529, -9.8322) centre (17.2645, -10.8143) ccw
  arc A387 (17.6546, -9.8935) -> (17.8445, -9.8277) centre (17.7131, -9.7554) ccw
  arc A388 (17.8445, -9.8277) -> (18.0853, -9.3772) centre (0, 0) ccw
  arc A389 (18.0853, -9.3772) -> (18.0345, -9.1827) centre (17.9522, -9.3081) ccw
  arc A390 (17.8714, -9.0491) -> (18.0345, -9.1827) centre (18.5834, -8.3468) ccw
  arc A391 (17.7821, -8.9408) -> (17.8714, -9.0491) centre (18.437, -8.4912) ccw
  arc A392 (17.7379, -8.3894) -> (17.7821, -8.9408) centre (18.2396, -8.6267) ccw
  arc A393 (18.1922, -8.0737) -> (17.7379, -8.3894) centre (18.2396, -8.6267) ccw
  arc A394 (18.3325, -8.0741) -> (18.1922, -8.0737) centre (18.2601, -8.8652) ccw
  arc A395 (18.5393, -8.1154) -> (18.3325, -8.0741) centre (18.2414, -9.07) ccw
  arc A396 (18.5393, -8.1154) -> (18.7219, -8.0313) centre (18.584, -7.9722) ccw
  arc A397 (18.7219, -8.0313) -> (18.9174, -7.5594) centre (0, 0) ccw
  arc A398 (18.9174, -7.5594) -> (18.8477, -7.3708) centre (18.7781, -7.5037) ccw
  arc A399 (18.6723, -7.2538) -> (18.8477, -7.3708) centre (19.312, -6.4851) ccw
  arc A400 (18.5728, -7.1548) -> (18.6723, -7.2538) centre (19.1805, -6.6432) ccw
  arc A401 (18.4748, -6.6104) -> (18.5728, -7.1548) centre (18.9974, -6.7974) ccw
  arc A402 (18.896, -6.2517) -> (18.4748, -6.6104) centre (18.9974, -6.7974) ccw
  arc A403 (19.0357, -6.2384) -> (18.896, -6.2517) centre (19.0411, -7.0327) ccw
  arc A404 (19.2455, -6.2592) -> (19.0357, -6.2384) centre (19.0425, -7.2383) ccw
  arc A405 (19.2455, -6.2592) -> (19.419, -6.1576) centre (19.276, -6.1123) ccw
  arc A406 (19.419, -6.1576) -> (19.5672, -5.6687) centre (0, 0) ccw
  arc A407 (19.5672, -5.6687) -> (19.4795, -5.4879) centre (19.4232, -5.627) ccw
  arc A408 (19.2934, -5.3886) -> (19.4795, -5.4879) centre (19.8547, -4.561) ccw
  arc A409 (19.1847, -5.2999) -> (19.2934, -5.3886) centre (19.7393, -4.7312) ccw
  arc A410 (19.0338, -4.7677) -> (19.1847, -5.2999) centre (19.5722, -4.9026) ccw
  arc A411 (19.4177, -4.3695) -> (19.0338, -4.7677) centre (19.5722, -4.9026) ccw
  arc A412 (19.5555, -4.3425) -> (19.4177, -4.3695) centre (19.6388, -5.1325) ccw
  arc A413 (19.7663, -4.3426) -> (19.5555, -4.3425) centre (19.6603, -5.337) ccw
  arc A414 (19.7663, -4.3426) -> (19.929, -4.2245) centre (19.7822, -4.1935) ccw
  arc A415 (19.929, -4.2245) -> (20.0287, -3.7235) centre (0, 0) ccw
  arc A416 (20.0287, -3.7235) -> (19.9236, -3.5522) centre (19.8812, -3.6961) ccw
  arc A417 (19.7287, -3.4716) -> (19.9236, -3.5522) centre (20.2061, -2.5929) ccw
  arc A418 (19.6118, -3.394) -> (19.7287, -3.4716) centre (20.108, -2.7736) ccw
  arc A419 (19.4095, -2.8791) -> (19.6118, -3.394) centre (19.9584, -2.9606) ccw
  arc A420 (19.7525, -2.4452) -> (19.4095, -2.8791) centre (19.9584, -2.9606) ccw
  arc A421 (19.887, -2.4048) -> (19.7525, -2.4452) centre (20.0473, -3.1828) ccw
  arc A422 (20.0968, -2.3843) -> (19.887, -2.4048) centre (20.0888, -3.3842) ccw
  arc A423 (20.0968, -2.3843) -> (20.2471, -2.2508) centre (20.098, -2.2343) ccw
  arc A424 (20.2471, -2.2508) -> (20.2972, -1.7424) centre (0, 0) ccw
  arc A425 (20.2972, -1.7424) -> (20.1758, -1.5822) centre (20.1477, -1.7296) ccw
  arc A426 (19.974, -1.5211) -> (20.1758, -1.5822) centre (20.363, -0.5999) ccw
  arc A427 (19.85, -1.4553) -> (19.974, -1.5211) centre (20.283, -0.7893) ccw
  arc A428 (19.5982, -0.9628) -> (19.85, -1.4553) centre (20.1525, -0.99) ccw
  arc A429 (19.8971, -0.4973) -> (19.5982, -0.9628) centre (20.1525, -0.99) ccw
  arc A430 (20.0269, -0.444) -> (19.8971, -0.4973) centre (20.2627, -1.2025) ccw
  arc A431 (20.2337, -0.403) -> (20.0269, -0.444) centre (20.3237, -1.3989) ccw
  arc A432 (20.2337, -0.403) -> (20.3702, -0.2554) centre (20.2202, -0.2536) ccw
  arc A433 (20.3702, -0.2554) -> (20.3702, 0.2554) centre (0, 0) ccw
  arc A434 (20.3702, 0.2554) -> (20.2337, 0.403) centre (20.2202, 0.2536) ccw
  arc A435 (20.0269, 0.444) -> (20.2337, 0.403) centre (20.3237, 1.3989) ccw
  arc A436 (19.8971, 0.4973) -> (20.0269, 0.444) centre (20.2627, 1.2025) ccw
  arc A437 (19.5982, 0.9628) -> (19.8971, 0.4973) centre (20.1525, 0.99) ccw
  arc A438 (19.85, 1.4553) -> (19.5982, 0.9628) centre (20.1525, 0.99) ccw
  arc A439 (19.974, 1.5211) -> (19.85, 1.4553) centre (20.283, 0.7893) ccw
  arc A440 (20.1758, 1.5822) -> (19.974, 1.5211) centre (20.363, 0.5999) ccw
  arc A441 (20.1758, 1.5822) -> (20.2972, 1.7424) centre (20.1477, 1.7296) ccw
  arc A442 (20.2972, 1.7424) -> (20.2471, 2.2508) centre (0, 0) ccw
  arc A443 (20.2471, 2.2508) -> (20.0968, 2.3843) centre (20.098, 2.2343) ccw
  arc A444 (19.887, 2.4048) -> (20.0968, 2.3843) centre (20.0888, 3.3842) ccw
  arc A445 (19.7525, 2.4452) -> (19.887, 2.4048) centre (20.0473, 3.1828) ccw
  arc A446 (19.4095, 2.8791) -> (19.7525, 2.4452) centre (19.9584, 2.9606) ccw
  arc A447 (19.6118, 3.394) -> (19.4095, 2.8791) centre (19.9584, 2.9606) ccw
  arc A448 (19.7287, 3.4716) -> (19.6118, 3.394) centre (20.108, 2.7736) ccw
  arc A449 (19.9236, 3.5522) -> (19.7287, 3.4716) centre (20.2061, 2.5929) ccw
  arc A450 (19.9236, 3.5522) -> (20.0287, 3.7235) centre (19.8812, 3.6961) ccw
  arc A451 (20.0287, 3.7235) -> (19.929, 4.2245) centre (0, 0) ccw
  arc A452 (19.929, 4.2245) -> (19.7663, 4.3426) centre (19.7822, 4.1935) ccw
  arc A453 (19.5555, 4.3425) -> (19.7663, 4.3426) centre (19.6603, 5.337) ccw
  arc A454 (19.4177, 4.3695) -> (19.5555, 4.3425) centre (19.6388, 5.1325) ccw
  arc A455 (19.0338, 4.7677) -> (19.4177, 4.3695) centre (19.5722, 4.9026) ccw
  arc A456 (19.1847, 5.2999) -> (19.0338, 4.7677) centre (19.5722, 4.9026) ccw
  arc A457 (19.2934, 5.3886) -> (19.1847, 5.2999) centre (19.7393, 4.7312) ccw
  arc A458 (19.4795, 5.4879) -> (19.2934, 5.3886) centre (19.8547, 4.561) ccw
  arc A459 (19.4795, 5.4879) -> (19.5672, 5.6687) centre (19.4232, 5.627) ccw
  arc A460 (19.5672, 5.6687) -> (19.419, 6.1576) centre (0, 0) ccw
  arc A461 (19.419, 6.1576) -> (19.2455, 6.2592) centre (19.276, 6.1123) ccw
  arc A462 (19.0357, 6.2384) -> (19.2455, 6.2592) centre (19.0425, 7.2383) ccw
  arc A463 (18.896, 6.2517) -> (19.0357, 6.2384) centre (19.0411, 7.0327) ccw
  arc A464 (18.4748, 6.6104) -> (18.896, 6.2517) centre (18.9974, 6.7974) ccw
  arc A465 (18.5728, 7.1548) -> (18.4748, 6.6104) centre (18.9974, 6.7974) ccw
  arc A466 (18.6723, 7.2538) -> (18.5728, 7.1548) centre (19.1805, 6.6432) ccw
  arc A467 (18.8477, 7.3708) -> (18.6723, 7.2538) centre (19.312, 6.4851) ccw
  arc A468 (18.8477, 7.3708) -> (18.9174, 7.5594) centre (18.7781, 7.5037) ccw
  arc A469 (18.9174, 7.5594) -> (18.7219, 8.0313) centre (0, 0) ccw
  arc A470 (18.7219, 8.0313) -> (18.5393, 8.1154) centre (18.584, 7.9722) ccw
  arc A471 (18.3325, 8.0741) -> (18.5393, 8.1154) centre (18.2414, 9.07) ccw
  arc A472 (18.1922, 8.0737) -> (18.3325, 8.0741) centre (18.2601, 8.8652) ccw
  arc A473 (17.7379, 8.3894) -> (18.1922, 8.0737) centre (18.2396, 8.6267) ccw
  arc A474 (17.7821, 8.9408) -> (17.7379, 8.3894) centre (18.2396, 8.6267) ccw
  arc A475 (17.8714, 9.0491) -> (17.7821, 8.9408) centre (18.437, 8.4912) ccw
  arc A476 (18.0345, 9.1827) -> (17.8714, 9.0491) centre (18.5834, 8.3468) ccw
  arc A477 (18.0345, 9.1827) -> (18.0853, 9.3772) centre (17.9522, 9.3081) ccw
  arc A478 (18.0853, 9.3772) -> (17.8445, 9.8277) centre (0, 0) ccw
  arc A479 (17.8445, 9.8277) -> (17.6546, 9.8935) centre (17.7131, 9.7554) ccw
  arc A480 (17.4529, 9.8322) -> (17.6546, 9.8935) centre (17.2645, 10.8143) ccw
  arc A481 (17.3132, 9.818) -> (17.4529, 9.8322) centre (17.3032, 10.6123) ccw
  arc A482 (16.8302, 10.0876) -> (17.3132, 9.818) centre (17.3062, 10.373) ccw
  arc A483 (16.8201, 10.6407) -> (16.8302, 10.0876) centre (17.3062, 10.373) ccw
  arc A484 (16.8984, 10.7572) -> (16.8201, 10.6407) centre (17.5159, 10.2575) ccw
  arc A485 (17.0476, 10.9062) -> (16.8984, 10.7572) centre (17.6758, 10.1281) ccw
  arc A486 (17.0476, 10.9062) -> (17.0791, 11.1047) centre (16.9534, 11.0229) ccw
  arc A487 (17.0791, 11.1047) -> (16.7953, 11.5295) centre (0, 0) ccw
  arc A488 (16.7953, 11.5295) -> (16.5999, 11.5763) centre (16.6716, 11.4446) ccw
  arc A489 (16.4051, 11.4955) -> (16.5999, 11.5763) centre (16.1214, 12.4544) ccw
  arc A490 (16.2675, 11.4677) -> (16.4051, 11.4955) centre (16.1797, 12.2572) ccw
  arc A491 (15.7604, 11.6887) -> (16.2675, 11.4677) centre (16.2062, 12.0193) ccw
  arc A492 (15.6961, 12.2381) -> (15.7604, 11.6887) centre (16.2062, 12.0193) ccw
  arc A493 (15.7627, 12.3617) -> (15.6961, 12.2381) centre (16.4262, 11.9249) ccw
  arc A494 (15.8965, 12.5247) -> (15.7627, 12.3617) centre (16.5979, 11.8119) ccw
  arc A495 (15.8965, 12.5247) -> (15.9084, 12.7253) centre (15.7913, 12.6316) ccw
  arc A496 (15.9084, 12.7253) -> (15.5844, 13.1202) centre (0, 0) ccw
  arc A497 (15.5844, 13.1202) -> (15.3853, 13.1476) centre (15.4696, 13.0236) ccw
  arc A498 (15.1994, 13.0481) -> (15.3853, 13.1476) centre (14.823, 13.9746) ccw
  arc A499 (15.0652, 13.007) -> (15.1994, 13.0481) centre (14.9004, 13.7841) ccw
  arc A500 (14.5388, 13.1772) -> (15.0652, 13.007) centre (14.95, 13.5499) ccw
  arc A501 (14.421, 13.7177) -> (14.5388, 13.1772) centre (14.95, 13.5499) ccw
  arc A502 (14.4751, 13.8472) -> (14.421, 13.7177) centre (15.1782, 13.4776) ccw
  arc A503 (14.5924, 14.0225) -> (14.4751, 13.8472) centre (15.3602, 13.3819) ccw
  arc A504 (14.5924, 14.0225) -> (14.5845, 14.2233) centre (14.4772, 14.1186) ccw
  arc A505 (14.5845, 14.2233) -> (14.2233, 14.5845) centre (0, 0) ccw
  arc A506 (14.2233, 14.5845) -> (14.0225, 14.5924) centre (14.1186, 14.4772) ccw
  arc A507 (13.8472, 14.4751) -> (14.0225, 14.5924) centre (13.3819, 15.3602) ccw
  arc A508 (13.7177, 14.421) -> (13.8472, 14.4751) centre (13.4776, 15.1782) ccw
  arc A509 (13.1772, 14.5388) -> (13.7177, 14.421) centre (13.5499, 14.95) ccw
  arc A510 (13.007, 15.0652) -> (13.1772, 14.5388) centre (13.5499, 14.95) ccw
  arc A511 (13.0481, 15.1994) -> (13.007, 15.0652) centre (13.7841, 14.9004) ccw
  arc A512 (13.1476, 15.3853) -> (13.0481, 15.1994) centre (13.9746, 14.823) ccw
  arc A513 (13.1476, 15.3853) -> (13.1202, 15.5844) centre (13.0236, 15.4696) ccw
  arc A514 (13.1202, 15.5844) -> (12.7253, 15.9084) centre (0, 0) ccw
  arc A515 (12.7253, 15.9084) -> (12.5247, 15.8965) centre (12.6316, 15.7913) ccw
  arc A516 (12.3617, 15.7627) -> (12.5247, 15.8965) centre (11.8119, 16.5979) ccw
  arc A517 (12.2381, 15.6961) -> (12.3617, 15.7627) centre (11.9249, 16.4262) ccw
  arc A518 (11.6887, 15.7604) -> (12.2381, 15.6961) centre (12.0193, 16.2062) ccw
  arc A519 (11.4677, 16.2675) -> (11.6887, 15.7604) centre (12.0193, 16.2062) ccw
  arc A520 (11.4955, 16.4051) -> (11.4677, 16.2675) centre (12.2572, 16.1797) ccw
  arc A521 (11.5763, 16.5999) -> (11.4955, 16.4051) centre (12.4544, 16.1214) ccw
  arc A522 (11.5763, 16.5999) -> (11.5295, 16.7953) centre (11.4446, 16.6716) ccw
  arc A523 (11.5295, 16.7953) -> (11.1047, 17.0791) centre (0, 0) ccw
  arc A524 (11.1047, 17.0791) -> (10.9062, 17.0476) centre (11.0229, 16.9534) ccw
  arc A525 (10.7572, 16.8984) -> (10.9062, 17.0476) centre (10.1281, 17.6758) ccw
  arc A526 (10.6407, 16.8201) -> (10.7572, 16.8984) centre (10.2575, 17.5159) ccw
  arc A527 (10.0876, 16.8302) -> (10.6407, 16.8201) centre (10.373, 17.3062) ccw
  arc A528 (9.818, 17.3132) -> (10.0876, 16.8302) centre (10.373, 17.3062) ccw
  arc A529 (9.8322, 17.4529) -> (9.818, 17.3132) centre (10.6123, 17.3032) ccw
  arc A530 (9.8935, 17.6546) -> (9.8322, 17.4529) centre (10.8143, 17.2645) ccw
  arc A531 (9.8935, 17.6546) -> (9.8277, 17.8445) centre (9.7554, 17.7131) ccw
  arc A532 (9.8277, 17.8445) -> (9.3772, 18.0853) centre (0, 0) ccw
  arc A533 (9.3772, 18.0853) -> (9.1827, 18.0345) centre (9.3081, 17.9522) ccw
  arc A534 (9.0491, 17.8714) -> (9.1827, 18.0345) centre (8.3468, 18.5834) ccw
  arc A535 (8.9408, 17.7821) -> (9.0491, 17.8714) centre (8.4912, 18.437) ccw
  arc A536 (8.3894, 17.7379) -> (8.9408, 17.7821) centre (8.6267, 18.2396) ccw
  arc A537 (8.0737, 18.1922) -> (8.3894, 17.7379) centre (8.6267, 18.2396) ccw